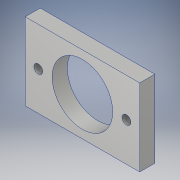
# Autodesk Inventor part: Tapered Roller Bearing Housing
Saved by Autodesk Inventor 2019 (Build 230136000, 136)
## iProperties
Created: 2018-11-13
Part Number: Tapered Roller Bearing Housing
Material: Aluminum 6061
Document SubType Name: Modeling
Designer: Alex Barnett
Density: 2.7 g/cm^3
Appearance: Aluminum - Flat
Author: Alex Barnett
Autodesk Inventor part; units mm, degrees
ref_plane "YZ Plane" through (0, 0, 0) normal (1, 0, 0) x (0, 1, 0)
ref_plane "XZ Plane" through (0, 0, 0) normal (0, 1, 0) x (-1, 0, 0)
ref_plane "XY Plane" through (0, 0, 0) normal (0, 0, 1) x (1, 0, 0)
sketch "Sketch1" plane through (0, 0, 0) normal (0, 0, 1) x (1, 0, 0)
  line L0 (-33.02, -22.225) -> (33.02, -22.225)
  line L1 (33.02, -22.225) -> (33.02, 22.225)
  line L2 (33.02, 22.225) -> (-33.02, 22.225)
  line L3 (-33.02, 22.225) -> (-33.02, -22.225)
  line L4 (-33.02, -22.225) -> (33.02, 22.225) construction
  line L5 (33.02, -22.225) -> (-33.02, 22.225) construction
  point P0 (0, 0)
  dimension "d0" = 66.04
  dimension "d1" = 44.45
  constraints: 12 end point, 2 midpoint, 2 parallel, 1 horizontal, 1 perpendicular
  measures "d0" distance of L2.end L1.end
  measures "d1" distance of L1.end L0.end
extrude "Extrusion1" add sketch "Sketch1" along normal mid plane 8.7376
sketch "Sketch2" plane through (0, 0, 4.3688) normal (0, 0, 1) x (1, 0, 0)
  line L0 (-33.02, -22.225) -> (33.02, -22.225) projected
  line L1 (33.02, -22.225) -> (33.02, 22.225) projected
  line L2 (33.02, 22.225) -> (-33.02, 22.225) projected
  line L3 (-33.02, 22.225) -> (-33.02, -22.225) projected
  circle A0 centre (0, 0) radius 17.4625
  dimension "d4" = 34.925
  constraints: 1 centre point, 1 coincident
  measures "d4" diameter of A0
hole "Hole1" at (0, 0, 4.3688) direction (0, 0, -1) diameter 34.925 end through all
sketch "Sketch3" plane through (0, 0, 4.3688) normal (0, 0, 1) x (1, 0, 0)
  circle A0 centre (0, 0) radius 17.4625 projected
  line L0 (-33.02, -22.225) -> (33.02, -22.225) projected
  line L1 (33.02, -22.225) -> (33.02, 22.225) projected
  line L2 (33.02, 22.225) -> (-33.02, 22.225) projected
  line L3 (-33.02, 22.225) -> (-33.02, -22.225) projected
  circle A1 centre (-25.4, 0) radius 2.54
  line L4 (0, 22.225) -> (0, -22.225) construction
  circle A2 centre (25.4, 0) radius 2.54
  dimension "d12" = 5.08
  dimension "d13" = 7.62
  constraints: 2 centre point, 2 end point, 2 midpoint, 1 symmetric about line, 1 other
  measures "d12" diameter of A1
  measures "d13" distance from line of L3 A1.centre
hole "Hole2" at (-25.4, 0, 4.3688) at (25.4, 0, 4.3688) direction (0, 0, -1) diameter 5.08 end through all
body "Solid1"
